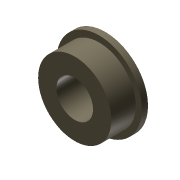
# Autodesk Inventor part: ベアリング(仮)
Saved by Autodesk Inventor 2011 SP1 (Build 150282100, 282)
## iProperties
Created: 2012-10-23
Part Number: ベアリング(仮)
Document SubType Name: Modeling
Designer: arihon
Density: 1 g/cm^3
Author: arihon
Autodesk Inventor part; units mm, degrees
ref_plane "YZ Plane" through (0, 0, 0) normal (1, 0, 0) x (0, 1, 0)
ref_plane "XZ Plane" through (0, 0, 0) normal (0, 1, 0) x (-1, 0, 0)
ref_plane "XY Plane" through (0, 0, 0) normal (0, 0, 1) x (1, 0, 0)
sketch "スケッチ1" plane through (0, 0, 0) normal (0, 0, 1) x (1, 0, 0)
  line L0 (-1.5, 2.9516) -> (-3, 2.9516)
  line L1 (-3, 2.9516) -> (-3, 0.4516)
  line L2 (-3, 0.4516) -> (-1.5, 0.4516)
  line L3 (-1.5, 0.4516) -> (-1.5, 2.9516)
  line L4 (-3, 2.9516) -> (-3.5, 2.9516)
  line L5 (-3.5, 2.9516) -> (-3.5, 2.4516)
  line L6 (-3.5, 2.4516) -> (-3, 2.4516)
  line L7 (-3, 2.4516) -> (-3, 2.9516)
  line L8 (0, 0) -> (0, 5.631)
  dimension "d0" = 1.5
  dimension "d1" = 3
  dimension "d2" = 2.5
  dimension "d3" = 3.5
  dimension "d4" = 0.5
  constraints: 18 end point, 5 parallel, 2 horizontal, 2 perpendicular
  measures "d0" distance from line of L8.start L3
  measures "d1" distance from line of L8.start L1
  measures "d2" distance of L2.end L0.start
  measures "d3" distance from line of L8.start L5
  measures "d4" distance of L4.end L5.end
revolve "回転1" add sketch "スケッチ1" angle 360 about axis through (0, 0, 0) along (0, 1, 0)
